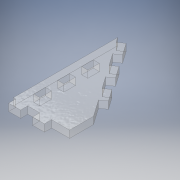
# Autodesk Inventor part: phone_holder_slider_side
Saved by Autodesk Inventor 2019 (Build 230136000, 136)
## iProperties
Created: 2019-02-17
Part Number: phone_holder_slider_side
Material: Acrylic, Clear
Document SubType Name: Modeling
Designer: suchanek
Density: 1.19 g/cm^3
Appearance: Transparent - Clear
Author: suchanek
Autodesk Inventor part; units mm, degrees
ref_plane "YZ Plane" through (0, 0, 0) normal (1, 0, 0) x (0, 1, 0)
ref_plane "XZ Plane" through (0, 0, 0) normal (0, 1, 0) x (-1, 0, 0)
ref_plane "XY Plane" through (0, 0, 0) normal (0, 0, 1) x (1, 0, 0)
sketch "Sketch2" plane through (0, 0, 0) normal (0, 1, 0) x (-1, 0, 0)
  line L0 (-23.5, 10) -> (23.5, 10)
  line L1 (23.5, 10) -> (23.5, -10)
  line L2 (23.5, -10) -> (17.5, -10)
  line L3 (-23.5, -10) -> (-23.5, 10)
  line L4 (-23.5, 10) -> (23.5, -10) construction
  line L5 (23.5, 10) -> (-23.5, -10) construction
  line L6 (21.5, 16) -> (11.5, 16)
  line L7 (11.5, 16) -> (11.5, 10)
  line L8 (11.5, 10) -> (21.5, 10)
  line L9 (21.5, 10) -> (21.5, 16)
  line L10 (-23.5, -10) -> (23.5, -77.123)
  line L11 (-23.5, -10) -> (58.442, -10) construction
  line L12 (23.5, -77.123) -> (23.5, -10)
  line L13 (20.6321, -73.0272) -> (13.7492, -63.1974)
  line L14 (13.7492, -63.1974) -> (8.8343, -66.6388)
  line L15 (8.8343, -66.6388) -> (15.7172, -76.4687)
  line L16 (15.7172, -76.4687) -> (20.6321, -73.0272)
  line L17 (6.8663, -53.3675) -> (-0.0166, -43.5377)
  line L18 (1.9514, -56.809) -> (6.8663, -53.3675)
  line L19 (-4.9315, -46.9792) -> (1.9514, -56.809)
  line L20 (-0.0166, -43.5377) -> (-4.9315, -46.9792)
  line L21 (-6.8996, -33.7079) -> (-13.7825, -23.8781)
  line L22 (-11.8145, -37.1494) -> (-6.8996, -33.7079)
  line L23 (-18.6974, -27.3195) -> (-11.8145, -37.1494)
  line L24 (-13.7825, -23.8781) -> (-18.6974, -27.3195)
  line L25 (1.5, 10) -> (-8.5, 10)
  line L26 (-8.5, 10) -> (-8.5, 16)
  line L27 (-8.5, 16) -> (1.5, 16)
  line L28 (1.5, 16) -> (1.5, 10)
  line L29 (-19.5182, -15.6866) -> (-23.5, -10)
  line L30 (-23.5, -10) -> (-28.4149, -13.4415)
  line L31 (-28.4149, -13.4415) -> (-24.4331, -19.128)
  line L32 (-24.4331, -19.128) -> (-19.5182, -15.6866)
  line L33 (17.5, -50.8098) -> (12.4, -50.8098)
  line L34 (12.4, -50.8098) -> (12.4, -41.1098)
  line L35 (12.4, -41.1098) -> (17.5, -41.1098)
  line L36 (17.5, -41.1098) -> (17.5, -50.8098)
  line L37 (17.5, -30.8098) -> (12.4, -30.8098)
  line L38 (17.5, -21.1098) -> (17.5, -30.8098)
  line L39 (12.4, -21.1098) -> (17.5, -21.1098)
  line L40 (12.4, -30.8098) -> (12.4, -21.1098)
  line L41 (17.5, -10.8098) -> (12.4, -10.8098)
  line L42 (17.5, -1.1098) -> (17.5, -10.8098)
  line L43 (12.4, -1.1098) -> (17.5, -1.1098)
  line L44 (12.4, -10.8098) -> (12.4, -1.1098)
  line L45 (12.4, -10) -> (-23.5, -10)
  line L46 (17.5, -10) -> (12.4, -10)
  point P0 (0, 0)
  dimension "d9" = 20
  dimension "d19" = 10
  dimension "d20" = 6
  dimension "d21" = 2
  dimension "d41" = 55
  dimension "d42" = 6
  dimension "d45" = 24
  dimension "d50" = 5
  dimension "d51" = 12
  dimension "d52" = 10
  dimension "d53" = 6
  dimension "d54" = 10
  dimension "d55" = 47
  dimension "d56" = 10
  dimension "d57" = 5.1
  dimension "d58" = 9.7
  dimension "d61" = 20
  dimension "d66" = 6
  dimension "d67" = 6
  constraints: 94 end point, 14 parallel, 8 point on line, 6 perpendicular, 5 horizontal, 3 collinear, 2 midpoint, 2 vertical, 1 equal length, 32 other
  measures "d9" distance of L0.end L1.end
  measures "d19" distance of L8.end L7.end
  measures "d20" distance of L7.end L6.end
  measures "d21" distance between parallel lines of L1 L9
  measures "d41" angle of L10 L11
  measures "d42" distance of L14.end L13.end
  measures "d45" distance of L13.end L17.end
  measures "d50" distance from line of L10.end L16
  measures "d51" distance of L14.end L15.end
  measures "d52" distance of L26.end L27.end
  measures "d53" distance of L25.end L26.end
  measures "d54" distance between parallel lines of L28 L7
  measures "d55" distance of L1.end L3.start
  measures "d56" distance between parallel lines of L32 L24
  measures "d57" distance of L34.end L35.end
  measures "d58" distance of L33.end L34.end
  measures "d61" distance of L33.start L37.start
  measures "d66" distance from line of L10 L33.end
  measures "d67" distance between parallel lines of L12 L36
extrude "Extrusion2" add sketch "Sketch2" along normal blind 6 contours L0 L1 L2 L42 L43 L44 L45 L3 | L26 L27 L28 L0 | L45 L44 L41 L42 L2 L12 L10 | L7 L6 L9 L0 | L10 L22 L23 L24 | L10 L18 L19 L20 | L16 L15 L14 L10
body "Solid2"
